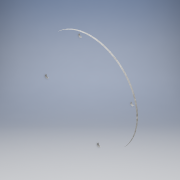
# Autodesk Inventor part: Light Sensor
Saved by Autodesk Inventor 2018 (Build 220112000, 112)
## iProperties
Created: 2018-09-04
Part Number: Light Sensor
Material: Generic
Document SubType Name: Modeling
Designer: matth
Density: 1 g/cm^3
Appearance: Default
Author: matth
Autodesk Inventor part; units mm, degrees
ref_plane "YZ Plane" through (0, 0, 0) normal (1, 0, 0) x (0, 1, 0)
ref_plane "XZ Plane" through (0, 0, 0) normal (0, 1, 0) x (-1, 0, 0)
ref_plane "XY Plane" through (0, 0, 0) normal (0, 0, 1) x (1, 0, 0)
sketch "Sketch1" plane through (0, 0, 0) normal (0, 1, 0) x (-1, 0, 0)
  circle A0 centre (0, 0) radius 45
  line L0 (0, 0) -> (0, -40.64)
  line L1 (0, -40.64) -> (-8.89, -40.64)
  circle A1 centre (-8.89, -40.64) radius 1.5
  circle A2 centre (40.64, -8.89) radius 1.5
  circle A3 centre (8.89, 40.64) radius 1.5
  circle A4 centre (-40.64, 8.89) radius 1.5
  dimension "d0" = 90
  dimension "d1" = 40.64
  dimension "d2" = 8.89
  dimension "d3" = 3
  dimension "d6" = 360
  constraints: 5 centre point, 4 end point, 2 coincident, 1 horizontal, 1 vertical, 9 other
  measures "d0" diameter of A0
  measures "d1" distance of L0.start L0.end
  measures "d2" distance of L0.end L1.end
  measures "d3" diameter of A1
extrude "Extrusion1" add sketch "Sketch1" along normal blind 1.5
sketch "Sketch2" plane through (0, 1.5, 0) normal (0, 1, 0) x (1, 0, 0)
  point P0 (0, 0)
body "Solid1"
